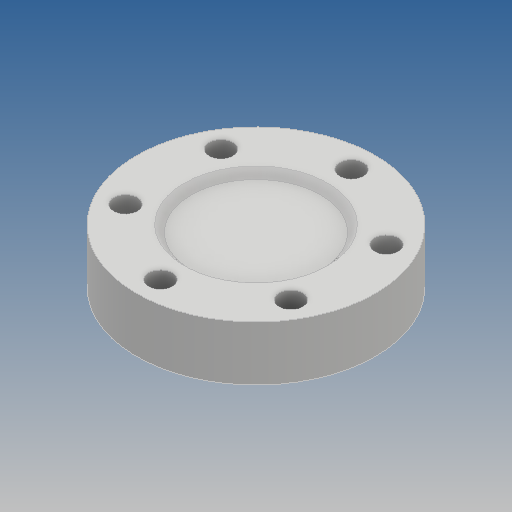
# Autodesk Inventor part: Flansch
Saved by Autodesk Inventor 2018 (Build 220112000, 112)
## iProperties
Created: 2018-09-25
Part Number: Flansch
Material: Generisch
Document SubType Name: Modeling
Designer: M.Knabel
Density: 1 g/cm^3
Appearance: Vorgabe
Mass: 6.75205 g
Surface Area: 34.3974 cm^2
Volume: 6.75205 cm^3
Author: M.Knabel
Autodesk Inventor part; units mm, degrees
ref_plane "XZ Plane" through (0, 0, 0) normal (0, 1, 0) x (-1, 0, 0)
ref_plane "XY Plane" through (0, 0, 0) normal (0, 0, 1) x (1, 0, 0)
sketch "Skizze1" plane through (0, 0, 0) normal (0, 0, 1) x (1, 0, 0)
  circle A0 centre (0, 0) radius 17.5
  line L0 (-24.5, 0) -> (24.5, 0) projected
  line L1 (0, -24.5) -> (0, 24.5) projected
  dimension "d0" = 35
  constraints: 1 centre point, 1 coincident
  measures "d0" diameter of A0
extrude "Extrusion1" add sketch "Skizze1" along normal blind 8
sketch "Skizze2" plane through (0, 0, 8) normal (0, 0, 1) x (1, 0, 0)
  line L0 (0, -24.5) -> (0, 24.5) projected
  line L1 (-24.5, 0) -> (24.5, 0) projected
  circle A0 centre (0, 0) radius 9.5
  dimension "d3" = 19
  constraints: 1 centre point, 1 coincident
  measures "d3" diameter of A0
extrude "Extrusion2" cut sketch "Skizze2" against normal blind 1
chamfer "Fase1" distance 1 angle 45 1 edges at (-9.5, 0, 8)
sketch "Skizze3" plane through (0, 0, 8) normal (0, 0, 1) x (1, 0, 0)
  line L0 (0, -24.5) -> (0, 24.5) projected
  line L1 (-24.5, 0) -> (24.5, 0) projected
  circle A0 centre (0, -14) radius 1.75
  point P0 (0, 0)
  dimension "d11" = 3.5
  dimension "d12" = 14
  constraints: 1 centre point, 1 point on line
  measures "d11" diameter of A0
  measures "d12" distance from line of L1 A0.centre
extrude "Extrusion3" cut sketch "Skizze3" against normal up to surface (8 mm away)
pattern_circular "Runde Anordnung1" count 6 over 360 about axis through (0, 0, 7.5) along (0, 0, 1) of "Extrusion3"
sketch "Skizze4" plane through (0, 0, 0) normal (0, 0, -1) x (-1, 0, 0)
  point P0 (0, 0)
  point P1 (0, 0)
  constraints: 1 coincident
hole "Bohrung1" at (0, 0, 0) direction (0, 0, 1) diameter 3 depth 5 tip angle 118
ref_plane "Arbeitsebene3" through (-17.5, 0, 0) normal (1, 0, 0) x (0, 1, 0)
sketch "Skizze7" plane through (-17.5, 0, 0) normal (1, 0, 0) x (0, 1, 0)
  line L0 (-24.5, 0) -> (24.5, 0) projected
  line L1 (0, -1.6) -> (0, 9.6) projected
  point P0 (0, 0)
  point P1 (0, 4)
  dimension "d28" = 4
  constraints: 1 midpoint
  measures "d28" distance from line of L0 point (0, 4)
hole "Bohrung2" at (-17.5, 0, 4) direction (1, 0, 0) diameter 3 depth 17.5 tip angle 118 counterbore diameter 4 counterbore depth 3
